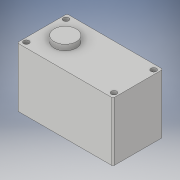
# Autodesk Inventor part: Servo_Block
Saved by Autodesk Inventor 2019 (Build 230136000, 136)
## iProperties
Created: 2021-02-23
Part Number: Servo_Block
Material: Generic
Document SubType Name: Modeling
Designer: zhanb
Density: 1 g/cm^3
Appearance: Default
Author: zhanb
Autodesk Inventor part; units mm, degrees
ref_plane "YZ Plane" through (0, 0, 0) normal (1, 0, 0) x (0, 1, 0)
ref_plane "XZ Plane" through (0, 0, 0) normal (0, 1, 0) x (-1, 0, 0)
ref_plane "XY Plane" through (0, 0, 0) normal (0, 0, 1) x (1, 0, 0)
sketch "Sketch1" plane through (0, 0, 0) normal (0, 1, 0) x (-1, 0, 0)
  line L0 (-22.01, 11.46) -> (22.01, 11.46)
  line L1 (22.01, 11.46) -> (22.01, -11.46)
  line L2 (22.01, -11.46) -> (-22.01, -11.46)
  line L3 (-22.01, -11.46) -> (-22.01, 11.46)
  line L4 (-22.01, 11.46) -> (22.01, -11.46) construction
  line L5 (22.01, 11.46) -> (-22.01, -11.46) construction
  line L6 (20.1, -9.1) -> (-20.1, -9.1) construction
  line L7 (-20.1, -9.1) -> (-20.1, 9.1) construction
  line L8 (-20.1, 9.1) -> (20.1, 9.1) construction
  line L9 (20.1, 9.1) -> (20.1, -9.1) construction
  line L10 (20.1, -9.1) -> (-20.1, 9.1) construction
  line L11 (-20.1, -9.1) -> (20.1, 9.1) construction
  circle A0 centre (11.35, 0) radius 5.08
  point P0 (0, 0)
  point P1 (22.01, 0)
  dimension "d0" = 18.2
  dimension "d1" = 40.2
  dimension "d2" = 44.02
  dimension "d3" = 22.92
  dimension "d4" = 33.36
  dimension "d5" = 10.16
  constraints: 24 end point, 5 midpoint, 4 coincident, 4 parallel, 2 horizontal, 2 perpendicular, 1 centre point, 1 horizontal alignment
  measures "d0" distance of L8.end L6.start
  measures "d1" distance of L7.end L8.end
  measures "d2" distance of L0.start L0.end
  measures "d3" distance of L0.end L1.end
  measures "d4" distance from line of L3 A0.centre
  measures "d5" diameter of A0
extrude "Extrusion1" add sketch "Sketch1" along normal mid plane 27 contours L0 L1 L2 L3 | A0
hole "Hole1" at (20.1, 0, -9.1) at (20.1, 0, 9.1) at (-20.1, 0, -9.1) at (-20.1, 0, 9.1) direction (0, 1, 0) diameter 2.5 end through all both
chamfer "Chamfer1" distance 0.5 angle 45 4 edges at (-22.01, 0, -11.46) (-22.01, 0, 11.46) (22.01, 0, -11.46) (22.01, 0, 11.46)
extrude "Extrusion2" add sketch "Sketch1" along normal mid plane 32.12 contours A0
body "Solid1"
